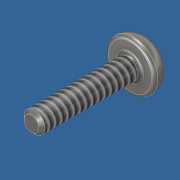
# Autodesk Inventor part: Screw
Saved by Autodesk Inventor 2018 (Build 220112000, 112)
## iProperties
Created: 2018-04-09
Part Number: Screw
Material: Stainless Steel
Document SubType Name: Modeling
Designer: 232963
Density: 8 g/cm^3
Appearance: Semi-Polished
Author: 232963
Autodesk Inventor part; units mm, degrees
ref_plane "YZ Plane" through (0, 0, 0) normal (1, 0, 0) x (0, 1, 0)
ref_plane "XZ Plane" through (0, 0, 0) normal (0, 1, 0) x (-1, 0, 0)
ref_plane "XY Plane" through (0, 0, 0) normal (0, 0, 1) x (1, 0, 0)
sketch "Sketch1" plane through (0, 0, 0) normal (0, 0, 1) x (1, 0, 0)
  circle A0 centre (0, 0) radius 1.0795
  dimension "d0" = 2.159
  constraints: 1 centre point, 1 coincident
  measures "d0" diameter of A0
extrude "Extrusion1" add sketch "Sketch1" along normal blind 10.16
sketch "Sketch2" plane through (0, 0, 0) normal (0, 0, -1) x (-1, 0, 0)
  circle A0 centre (0, 0) radius 2.54
  dimension "d3" = 5.08
  constraints: 1 centre point, 1 coincident
  measures "d3" diameter of A0
extrude "Extrusion2" add sketch "Sketch2" along normal blind 1.905
fillet "Fillet1" radius 1.5875 1 edges at (2.54, 0, -1.905)
fillet "Fillet2" radius 0.3175 1 edges at (-1.0795, 0, 0)
fillet "Fillet3" radius 0.3175 1 edges at (2.54, 0, 0)
chamfer "Chamfer1" distance 0.3175 angle 45 1 edges at (-1.0795, 0, 10.16)
sketch "Sketch3" plane through (0, 0, -1.905) normal (0, 0, -1) x (-1, 0, 0)
  line L0 (-1.3748, 0) -> (-0.6874, 1.1906)
  line L1 (-0.6874, 1.1906) -> (0.6874, 1.1906)
  line L2 (0.6874, 1.1906) -> (1.3748, 0)
  line L3 (1.3748, 0) -> (0.6874, -1.1906)
  line L4 (0.6874, -1.1906) -> (-0.6874, -1.1906)
  line L5 (-0.6874, -1.1906) -> (-1.3748, 0)
  point P0 (0, 0)
  point P1 (0, 0)
  dimension "d17" = 2.3813
  constraints: 12 end point, 1 coincident, 13 other
  measures "d17" distance between parallel lines of L4 L1
extrude "Extrusion3" cut sketch "Sketch3" against normal blind 0.635
thread "Thread1" size "4-40 UNC" class "2A" standard "ANSI Unified Screw Threads" full length
body "Solid1"
